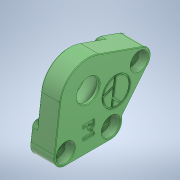
# Autodesk Inventor part: X-Axis Motor Support
Saved by Autodesk Inventor 2020 (Build 240168000, 168)
## iProperties
Created: 2019-09-17
Part Number: X-Axis Motor Support
Material: Generic
Document SubType Name: Modeling
Designer: pepd9
Density: 1 g/cm^3
Appearance: Smooth - Dark Forest Green
Author: pepd9
Autodesk Inventor part; units mm, degrees
ref_plane "YZ Plane" through (0, 0, 0) normal (1, 0, 0) x (0, 1, 0)
ref_plane "XZ Plane" through (0, 0, 0) normal (0, 1, 0) x (-1, 0, 0)
ref_plane "XY Plane" through (0, 0, 0) normal (0, 0, 1) x (1, 0, 0)
sketch "Sketch1" plane through (0, 0, 0) normal (1, 0, 0) x (0, 1, 0)
  circle A0 centre (0, 0) radius 8
  circle A1 centre (0, 0) radius 10
  dimension "d0" = 16
  dimension "d1" = 20
  constraints: 2 centre point, 2 coincident
  measures "d0" diameter of A0
  measures "d1" diameter of A1
extrude "Extrusion1" add sketch "Sketch1" along normal blind 6
sketch "Sketch2" plane through (0, 0, 0) normal (-1, 0, 0) x (0, 0, 1)
  circle A0 centre (0, 0) radius 8
  circle A1 centre (-18, 0) radius 2.75 construction
  circle A2 centre (-18, 0) radius 4
  circle A3 centre (0, 0) radius 10
  circle A4 centre (-18, 0) radius 1.5 construction
  line L0 (-19.5, 3.708099) -> (-3.736025, 9.275889)
  circle A5 centre (0, 0) radius 10
  line L1 (-12.888145, -9.569739) -> (-10.705089, -10.830127) construction
  line L2 (10.373932, -10.830127) -> (12.998008, -9.315116) construction
  circle A6 centre (-8, -15) radius 1.5 construction
  circle A7 centre (8, -15) radius 1.5 construction
  circle A8 centre (8, -15) radius 2.75 construction
  circle A9 centre (-8, -15) radius 2.75 construction
  circle A10 centre (-8, -15) radius 4
  circle A11 centre (8, -15) radius 4
  line L3 (-12, -15) -> (-12, -13.5)
  line L4 (11.832818, -13.855665) -> (9.920905, 1.255246)
  line L5 (8, -19) -> (-8, -19)
  line L6 (-12, -13.5) -> (-20.414736, -3.188895)
  point P0 (9.920905, 1.255246)
  point P1 (-3.736025, 9.275889)
  dimension "d4" = 5.5
  dimension "d5" = 8
  dimension "d6" = 18
  dimension "d7" = 3
  dimension "d8" = 3
  dimension "d9" = 3
  dimension "d10" = 5.5
  dimension "d11" = 5.5
  dimension "d12" = 8
  dimension "d13" = 8
  dimension "d14" = 15
  dimension "d15" = 8
  dimension "d16" = 8
  constraints: 10 end point, 9 centre point, 9 coincident, 8 point on circle, 2 tangent, 1 horizontal alignment, 1 vertical
  measures "d4" diameter of A1
  measures "d5" diameter of A2
  measures "d6" distance of point (0, 0) A1.centre
  measures "d7" diameter of A4
  measures "d8" diameter of A6
  measures "d9" diameter of A7
  measures "d10" diameter of A8
  measures "d11" diameter of A9
  measures "d12" diameter of A10
  measures "d13" diameter of A11
  measures "d14" vertical distance of A6.centre point (0, 0)
  measures "d15" horizontal distance of point (0, 0) A8.centre
  measures "d16" horizontal distance of point (0, 0) A6.centre
extrude "Extrusion2" add sketch "Sketch2" against normal blind 6 contours A2 | A2 L0 A3 L4 A11 L5 A10 L3 L6 | A10 | A11
sketch "Sketch3" plane through (6, 0, 0) normal (1, 0, 0) x (0, 0, -1)
  arc A0 (20.414736, -3.188895) -> (19.5, 3.708099) centre (18, 0) ccw
  arc A1 (8, -19) -> (12, -15) centre (8, -15) ccw
  arc A2 (-11.832818, -13.855665) -> (-8, -19) centre (-8, -15) ccw
  point P0 (0, 0)
hole "Hole1" at (6, 0, -18) at (6, -15, -8) at (6, -15, 8) direction (-1, 0, 0) diameter 3.2 end through all counterbore diameter 6.5 counterbore depth 2 clearance for "Socket Head Cap Screw" size "M3" standard "Ansi Metric M Profile"
sketch "Sketch4" plane through (6, 0, 0) normal (1, 0, 0) x (0, 0, -1)
  circle A0 centre (8, -15) radius 3.25
  circle A1 centre (18, 0) radius 3.25
  circle A2 centre (-8, -15) radius 3.25
  arc A3 (3.736025, 9.275889) -> (-9.920905, 1.255246) centre (0, 0) ccw
  line L0 (-9.920905, 1.255246) -> (-11.832818, -13.855665)
  arc A4 (-11.832818, -13.855665) -> (-8, -19) centre (-8, -15) ccw
  line L1 (-8, -19) -> (8, -19)
  arc A5 (8, -19) -> (12, -15) centre (8, -15) ccw
  line L2 (12, -15) -> (12, -13.5)
  line L3 (12, -13.5) -> (20.414736, -3.188895)
  arc A6 (20.414736, -3.188895) -> (19.5, 3.708099) centre (18, 0) ccw
  line L4 (19.5, 3.708099) -> (3.736025, 9.275889)
  circle A7 centre (0, 0) radius 8
  circle A8 centre (0, 0) radius 4
  dimension "d26" = 8
  constraints: 1 centre point, 1 coincident
  measures "d26" diameter of A8
extrude "Extrusion3" add sketch "Sketch4" along normal blind 1 contours L4 A6 L3 L2 A5 L1 A4 L0 A3 | A7
sketch "Sketch5" plane through (0, 0, 0) normal (-1, 0, 0) x (0, 0, 1)
  circle A0 centre (-8, -15) radius 1.6
  circle A1 centre (-18, 0) radius 1.6
  circle A2 centre (8, -15) radius 1.6
  arc A3 (9.920905, 1.255246) -> (-3.736025, 9.275889) centre (0, 0) ccw
  line L0 (-3.736025, 9.275889) -> (-19.5, 3.708099)
  arc A4 (-19.5, 3.708099) -> (-20.414736, -3.188895) centre (-18, 0) ccw
  line L1 (-20.414736, -3.188895) -> (-12, -13.5)
  line L2 (-12, -13.5) -> (-12, -15)
  arc A5 (-12, -15) -> (-8, -19) centre (-8, -15) ccw
  line L3 (-8, -19) -> (8, -19)
  arc A6 (8, -19) -> (11.832818, -13.855665) centre (8, -15) ccw
  line L4 (11.832818, -13.855665) -> (9.920905, 1.255246)
  circle A7 centre (0, 0) radius 8
  circle A8 centre (0, 0) radius 8
  line L5 (0, -8) -> (11.091928, -8)
  line L6 (11.832818, -13.855665) -> (9.920905, 1.255246)
  line L7 (-7.667515, -2.282371) -> (-10.979812, 6.717405)
  constraints: 4 end point, 2 point on circle, 2 point on line, 1 horizontal, 1 tangent
ref_plane "Work Plane1" through (-3.5, -20.915116, -29.665578) normal (1, 0, 0) x (0, 1, 0)
extrude "Extrusion4" add sketch "Sketch5" along normal blind 1.8 contours L4 A6 L3 A5 L2 L1 A4 L0 L7 A7 L5
fillet "Fillet1" radius 2 2 edges at (-0.9, -8, 11.0919) (-0.9, 6.7174, -10.9798)
chamfer "Chamfer1" distance 0.5 angle 45 13 edges at (-1.8, 0.5259, -21.9653) (-1.8, 4.8841, -16.1705) (-1.8, 5.9843, -11.3243) (-1.8, 1.2913, -8.9828) (-1.8, -6.4132, -4.7823) (-1.8, -8, 4.6645) (-1.8, -8.4997, 10.6515) (-1.8, -11.8023, 11.573) (-1.8, -17.3898, 11.2076) (-1.8, -19, 0) (-1.8, -17.8284, -10.8284) (-1.8, -14.25, -12) (-1.8, -8.3444, -16.2074)
chamfer "Chamfer2" distance 0.2 angle 45 12 edges at (7, 8.6229, 5.0642) (7, -6.3002, 10.8769) (7, 6.492, -11.618) (7, 0.5259, -21.9653) (7, -8.3444, -16.2074) (7, -17.8284, -10.8284) (7, -14.25, -12) (7, -19, 0) (7, -17.3898, 11.2076) (7, -15, 11.25) (7, 0, 4) (7, -15, -4.75)
chamfer "Chamfer3" distance 0.5 angle 45 5 edges at (0, -3.3724, 10.5064) (0, -8.8745, 11.2026) (0, 8.6229, 5.0642) (0, 7.9966, -7.3579) (0, 6.3887, -11.9104)
chamfer "Chamfer4" distance 0.5 angle 45 2 edges at (0, 4.7823, -6.4132) (0, 0, 8)
sketch "Sketch6" plane through (7, 0, 0) normal (1, 0, 0) x (0, 0, -1)
  line L0 (2.0671, -9.323665) -> (2.0671, -25.516059) construction
  line L1 (2.0671, -25.516059) -> (-8.9329, -25.516059) construction
  line L2 (-8.9329, -25.516059) -> (-8.9329, -9.323665) construction
  line L3 (-8.9329, -9.323665) -> (2.0671, -9.323665) construction
  circle A0 centre (9.780392, -5.00002) radius 5
  circle A1 centre (9.780392, -5.00002) radius 4.5
  line L4 (9.780392, -0.50002) -> (8.53296, -9.323665)
  line L5 (9.168517, -0.541813) -> (7.956649, -9.113894)
  line L6 (8.9452, -6.407706) -> (11.604135, -9.113894)
  line L7 (8.839394, -7.15612) -> (10.981861, -9.336663)
  line L8 (8.841937, -2.851862) -> (5.352705, -4.196537)
  line L9 (8.745793, -3.531927) -> (5.282369, -4.866656)
  line L10 (-1.9329, -9.53843) -> (2.0671, -9.53843)
  line L11 (2.0671, -9.53843) -> (2.0671, -11.09846)
  spline S0 degree 2 poles (2.0671, -11.09846) (2.0671, -11.641339) (1.592827, -12.205097) (1.08276, -12.288617) knots 0 0 0 1 2 2 2
  spline S1 degree 2 poles (1.08276, -12.288617) (0.915721, -12.31248) (0.79939, -12.318445) (0.754647, -12.318445) knots 0 0 0 1 2 2 2
  spline S2 degree 2 poles (0.754647, -12.318445) (0.190889, -12.318445) (-0.441475, -11.620459) (-0.441475, -10.997043) knots 0 0 0 1 2 2 2
  line L12 (-0.441475, -10.997043) -> (-0.441475, -10.680861)
  line L13 (-0.441475, -10.680861) -> (-1.9329, -10.680861)
  line L14 (-1.9329, -10.680861) -> (-1.9329, -9.53843)
  spline S3 degree 2 poles (0.399688, -10.850884) (0.399688, -10.934403) (0.539882, -11.113374) (0.683059, -11.143203) knots 0 0 0 1 2 2 2
  spline S4 degree 2 poles (0.683059, -11.143203) (0.75763, -11.158117) (0.823253, -11.158117) knots 0 0 0 1 1 1
  spline S5 degree 2 poles (0.823253, -11.158117) (1.008189, -11.158117) (1.219971, -10.985112) (1.219971, -10.862815) knots 0 0 0 1 2 2 2
  line L15 (1.219971, -10.862815) -> (1.219971, -10.680861)
  line L16 (1.219971, -10.680861) -> (0.399688, -10.680861)
  line L17 (0.399688, -10.680861) -> (0.399688, -10.850884)
  line L18 (0.71587, -12.566022) -> (1.494393, -12.566022)
  line L19 (1.494393, -12.566022) -> (1.488428, -12.718147)
  line L20 (1.488428, -12.718147) -> (1.503342, -12.923964)
  spline S6 degree 2 poles (1.503342, -12.923964) (1.536153, -13.210317) (1.715124, -13.478773) (1.911992, -13.565276) knots 0 0 0 1 2 2 2
  line L21 (1.911992, -13.565276) -> (2.0671, -13.607036)
  line L22 (2.0671, -13.607036) -> (2.0671, -14.406439)
  line L23 (2.0671, -14.406439) -> (-1.9329, -14.406439)
  line L24 (-1.9329, -14.406439) -> (-1.9329, -13.278923)
  line L25 (-1.9329, -13.278923) -> (0.71587, -13.278923)
  line L26 (0.71587, -13.278923) -> (0.71587, -12.566022)
  point P0 (0, 0)
  dimension "d44" = 10
  dimension "d45" = 0.5
  dimension "d46" = 0.6
  dimension "d47" = 0.6
  dimension "d48" = 0.6
  constraints: 12 end point, 4 point on line, 3 parallel, 1 centre point, 12 other
  measures "d44" diameter of A0
  measures "d46" distance between parallel lines of L4 L5
  measures "d47" distance between parallel lines of L6 L7
  measures "d48" distance between parallel lines of L9 L8
extrude "Extrusion5" cut sketch "Sketch6" against normal blind 0.4 contours A0 | L4 A1 L5 | A1 L7 L4 L6 | L8 L5 L9 A1 | L10 L11 S0 S1 S2 L12 L13 L14 | L18 L19 L20 S6 L21 L22 L23 L24 L25 L26
sketch "Sketch7" plane through (4, 0, -18) normal (1, 0, 0) x (0, 0, -1)
  circle A0 centre (0, 0) radius 3.25 projected
  circle A1 centre (0, 0) radius 1.6 projected
  circle A2 centre (-10, -15) radius 3.25 projected
  circle A3 centre (-10, -15) radius 1.6 projected
  circle A4 centre (-26, -15) radius 3.25 projected
  circle A5 centre (-26, -15) radius 1.6 projected
  line L0 (-3.25, 1.6) -> (3.25, 1.6)
  line L1 (3.25, 1.6) -> (3.25, -1.6)
  line L2 (3.25, -1.6) -> (-3.25, -1.6)
  line L3 (-3.25, -1.6) -> (-3.25, 1.6)
  line L4 (-3.25, 1.6) -> (3.25, -1.6) construction
  line L5 (3.25, 1.6) -> (-3.25, -1.6) construction
  line L6 (-13.25, -13.4) -> (-6.75, -13.4)
  line L7 (-6.75, -13.4) -> (-6.75, -16.6)
  line L8 (-6.75, -16.6) -> (-13.25, -16.6)
  line L9 (-13.25, -16.6) -> (-13.25, -13.4)
  line L10 (-13.25, -13.4) -> (-6.75, -16.6) construction
  line L11 (-6.75, -13.4) -> (-13.25, -16.6) construction
  line L12 (-29.25, -13.4) -> (-22.75, -13.4)
  line L13 (-22.75, -13.4) -> (-22.75, -16.6)
  line L14 (-22.75, -16.6) -> (-29.25, -16.6)
  line L15 (-29.25, -16.6) -> (-29.25, -13.4)
  line L16 (-29.25, -13.4) -> (-22.75, -16.6) construction
  line L17 (-22.75, -13.4) -> (-29.25, -16.6) construction
  point P0 (-18, 0)
  point P1 (-26, -16.6)
  point P2 (-23.171131, -16.6)
  point P3 (-23.171131, -13.4)
  point P4 (-26, -13.4)
  point P5 (-28.828869, -16.6)
  point P6 (-28.828869, -13.4)
  point P7 (-10, -16.6)
  point P8 (-7.171131, -16.6)
  point P9 (-7.171131, -13.4)
  point P10 (-10, -13.4)
  point P11 (-12.828869, -16.6)
  point P12 (-12.828869, -13.4)
  point P13 (-2.828869, -1.6)
  point P14 (0, -1.6)
  point P15 (0, 1.6)
  point P16 (-2.828869, 1.6)
  point P17 (2.828869, -1.6)
  point P18 (2.828869, 1.6)
  constraints: 36 end point, 6 midpoint, 6 parallel, 3 horizontal, 3 perpendicular
extrude "Extrusion6" cut sketch "Sketch7" against normal blind 0.4 contours A0 L2 A1 L0 | L0 A1 L2 A0 | A2 L8 A3 L6 | L6 A3 L8 A2 | A4 L14 A5 L12 | L12 A5 L14 A4
body "Solid1"
